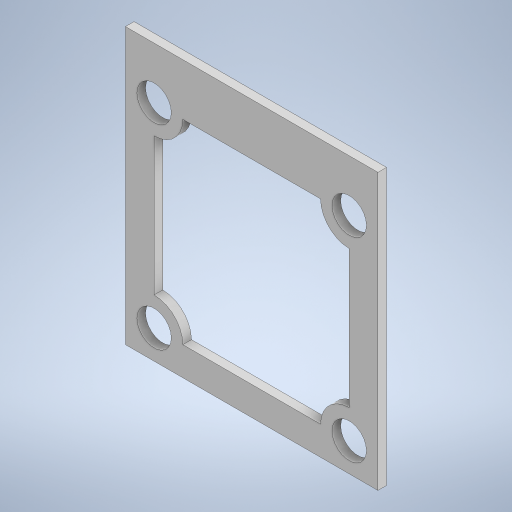
# Autodesk Inventor part: board_setter_base
Saved by Autodesk Inventor 2024.1 (Build 281209000, 209)
## iProperties
Created: 2024-10-09
Part Number: board_setter_base
Material: 一般
Document SubType Name: Sheet Metal
Designer: hibik
Density: 1 g/cm^3
Sheet Metal Rule: Default_mm
Appearance: 既定
Author: hibik
Autodesk Inventor part; units mm, degrees
ref_plane "YZ Plane" through (0, 0, 0) normal (1, 0, 0) x (0, 1, 0)
ref_plane "XZ Plane" through (0, 0, 0) normal (0, 1, 0) x (-1, 0, 0)
ref_plane "XY Plane" through (0, 0, 0) normal (0, 0, 1) x (1, 0, 0)
sketch "スケッチ1" plane through (0, 0, 0) normal (0, 0, 1) x (1, 0, 0)
  line L0 (-22, -24) -> (22, -24)
  line L1 (22, -24) -> (22, 24)
  line L2 (22, 24) -> (-22, 24)
  line L3 (-22, 24) -> (-22, -24)
  line L4 (-22, -24) -> (22, 24) construction
  line L5 (22, -24) -> (-22, 24) construction
  line L6 (-17, 15) -> (17, 15)
  line L7 (17, 15) -> (17, -19)
  line L8 (17, -19) -> (-17, -19)
  line L9 (-17, -19) -> (-17, 15)
  circle A0 centre (-17, 15) radius 3
  circle A1 centre (17, 15) radius 3
  circle A2 centre (17, -19) radius 3
  circle A3 centre (-17, -19) radius 3
  circle A4 centre (-17, 15) radius 5
  circle A5 centre (17, 15) radius 5
  circle A6 centre (17, -19) radius 5
  circle A7 centre (-17, -19) radius 5
  point P0 (0, 0)
  point P1 (-12, 15)
  point P2 (12, 15)
  point P3 (17, 10)
  point P4 (17, -14)
  point P5 (12, -19)
  point P6 (-12, -19)
  point P7 (-17, -14)
  point P8 (-17, 10)
  dimension "d0" = 48
  dimension "d1" = 44
  dimension "d2" = 34
  dimension "d3" = 5
  dimension "d4" = 5
  dimension "d5" = 6
  dimension "d6" = 10
  dimension "d7" = 10
  dimension "d8" = 10
  dimension "d9" = 10
  measures "d0" distance of L2.end L0.start
  measures "d1" distance of L1.end L2.end
  measures "d2" distance of L7.end L8.end
  measures "d3" distance between parallel lines of L3 L9
  measures "d4" distance between parallel lines of L0 L8
  measures "d5" diameter of A0
  measures "d6" diameter of A4
  measures "d7" diameter of A5
  measures "d8" diameter of A6
  measures "d9" diameter of A7
extrude "プレート1" add sketch "スケッチ1" along normal blind 1.5 contours L3 A7 L0 | A7 L8 A6 L0 | A7 L9 A3 L8 | L3 A4 L9 A7 | A6 L1 L0 | A6 L8 A2 L7 | L8 A3 L9 A7 | L3 L2 L1 A5 L6 A4 | A4 L6 A0 L9 | A6 L7 A2 L8 | A6 L7 A5 L1 | A4 L9 A0 L6 | A5 L7 A1 L6 | L6 A1 L7 A5
equation "\"d4\" = d3"
equation "\"d10\" = Thickness"
equation "\"BendRadius\" = Thickness"
equation "\"BendReliefWidth\" = Thickness"
equation "\"BendReliefDepth\" = 0.5 * Thickness"
equation "\"CornerReliefSize\" = 4 * Thickness"
equation "\"MinimumRemnant\" = 2 * Thickness"
equation "\"TransitionRadius\" = BendRadius"
equation "\"JacobiRadiusSize\" = BendRadius"
equation "\"GapSize\" = Thickness"
equation "\"Thickness\" = 1.5"
